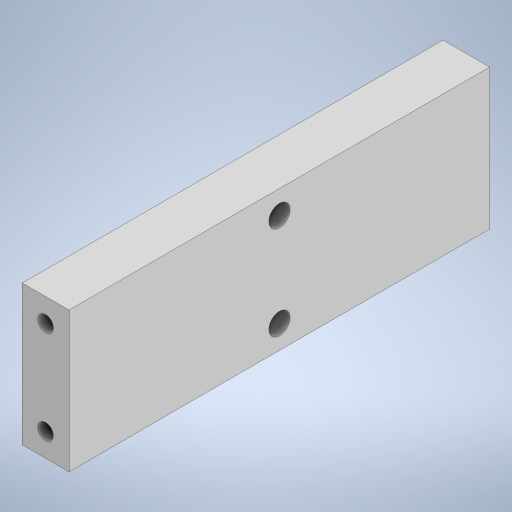
# Autodesk Inventor part: base_part_attachment_ver2
Saved by Autodesk Inventor 2024.3 (Build 283343000, 343)
## iProperties
Created: 2024-10-09
Part Number: base_part_attachment_ver2
Material: 一般
Document SubType Name: Modeling
Designer: hikou
Density: 1 g/cm^3
Appearance: 既定
Author: hikou
Autodesk Inventor part; units mm, degrees
ref_plane "YZ Plane" through (0, 0, 0) normal (1, 0, 0) x (0, 1, 0)
ref_plane "XZ Plane" through (0, 0, 0) normal (0, 1, 0) x (-1, 0, 0)
ref_plane "XY Plane" through (0, 0, 0) normal (0, 0, 1) x (1, 0, 0)
sketch "スケッチ1" plane through (0, 0, 0) normal (0, 0, 1) x (1, 0, 0)
  line L0 (-5, -15) -> (5, -15)
  line L1 (5, -15) -> (5, 15)
  line L2 (5, 15) -> (-5, 15)
  line L3 (-5, 15) -> (-5, -15)
  line L4 (-5, -15) -> (5, 15) construction
  line L5 (5, -15) -> (-5, 15) construction
  point P0 (0, 0)
  dimension "d0" = 10
  dimension "d1" = 30
  constraints: 12 end point, 2 midpoint, 2 parallel, 1 horizontal, 1 perpendicular
  measures "d0" distance of L2.end L1.end
  measures "d1" distance of L0.end L1.end
extrude "押し出し1" add sketch "スケッチ1" along normal mid plane 90
sketch "スケッチ2" plane through (0, 0, 45) normal (0, 0, 1) x (1, 0, 0)
  line L0 (5, 15) -> (-5, 15) projected
  line L1 (5, -15) -> (5, 15) projected
  line L2 (-5, -15) -> (5, -15) projected
  point P0 (0, 0)
  point P1 (0, 10)
  point P2 (0, -10)
  dimension "d4" = 5
  dimension "d5" = 5
  dimension "d6" = 5
  dimension "d7" = 5
  measures "d4" distance from line of L0 point (0, 10)
  measures "d5" distance from line of L1 point (0, 10)
  measures "d6" distance from line of L1 point (0, -10)
  measures "d7" distance from line of L2 point (0, -10)
hole "穴1" at (0, 10, 45) at (0, -10, 45) direction (0, 0, -1) diameter 3.3 depth 10 tip angle 118
sketch "スケッチ3" plane through (0, 0, -45) normal (0, 0, -1) x (-1, 0, 0)
  circle A0 centre (0, 10) radius 1.65 projected
  circle A1 centre (0, -10) radius 1.65 projected
  point P0 (0, 0)
  constraints: 2 coincident
hole "穴2" at (0, 10, -45) at (0, -10, -45) direction (0, 0, 1) diameter 3.3 depth 10 tip angle 118
sketch "スケッチ4" plane through (5, -15, 45) normal (1, 0, 0) x (0, 0, -1)
  line L0 (90, 30) -> (0, 30) projected
  line L1 (0, 0) -> (0, 30) projected
  point P0 (45, 15)
  point P1 (45, 25)
  point P2 (45, 5)
  point P3 (45, 30)
  dimension "d22" = 5
  dimension "d23" = 20
  dimension "d24" = 45
  dimension "d25" = 45
  constraints: 1 midpoint
  measures "d22" distance of point (45, 30) point (45, 25)
  measures "d23" distance of point (45, 5) point (45, 25)
  measures "d24" distance from line of L1 point (45, 25)
  measures "d25" distance from line of L1 point (45, 5)
hole "穴3" at (5, 10, 0) at (5, -10, 0) direction (-1, 0, 0) diameter 4.5 end through all
equation "\"d5\" = d4"
equation "\"d6\" = d4"
equation "\"d7\" = d4"
equation "\"d25\" = d24"
